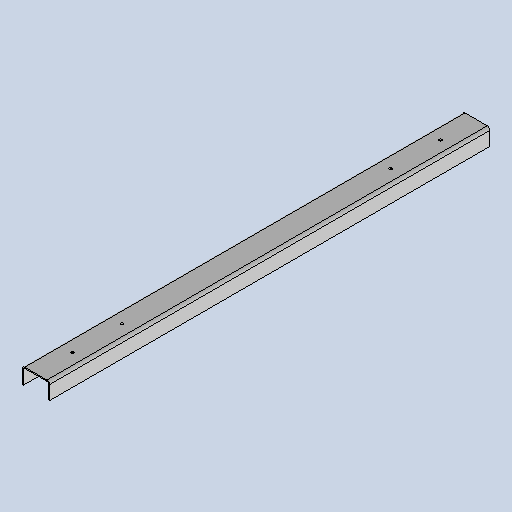
# Autodesk Inventor part: ДМФ 053 швеллер лотка v2.0_CPY
Saved by Autodesk Inventor 2026.2 (Build 302298010, 298A)
## iProperties
Created: 2024-05-13
Part Number: ДМФ 053 швеллер лотка v2.0_CPY
Material: Generic
Document SubType Name: Sheet Metal
Designer: admin
Mass: 164.292 g
Surface Area: 1680.29 cm^2
Volume: 164.292 cm^3
Density: 1 g/cm^3
Flat Pattern Width: 80 cm
Flat Pattern Length: 10.2404 cm
Flat Pattern Area: 819.232 cm^2
Sheet Metal Rule: Default
Sheet Metal Width: 800,000 mm
Sheet Metal Length: 102,404 mm
Sheet Metal Area: 81923,185 mm^2
Appearance: Default
Author: admin
Autodesk Inventor part; units mm, degrees
ref_plane "YZ Plane" through (0, 0, 0) normal (1, 0, 0) x (0, 1, 0)
ref_plane "XZ Plane" through (0, 0, 0) normal (0, 1, 0) x (-1, 0, 0)
ref_plane "XY Plane" through (0, 0, 0) normal (0, 0, 1) x (1, 0, 0)
sketch "Sketch1" plane through (0, 0, 0) normal (0, 0, 1) x (1, 0, 0)
  line L0 (-25, 0) -> (25, 0)
  line L1 (25, 0) -> (25, -800)
  line L2 (25, -800) -> (-25, -800)
  line L3 (-25, -800) -> (-25, 0)
  point P0 (0, 0)
  point P1 (0, 0)
  dimension "d0" = 50
  dimension "d1" = 800
  measures "d0" distance of L1.end L2.end
  measures "d1" distance of L0.end L1.end
extrude "Plate1" add sketch "Sketch1" along normal blind 2
sketch "Sketch2" plane through (23, -800, 2) normal (1, 0, 0) x (0, 1, 0)
  line L0 (800, 0) -> (0, 0)
  line L1 (0, 0) -> (0, -30)
  line L2 (0, -30) -> (800, -30)
  line L3 (800, -30) -> (800, 0)
  constraints: 6 end point, 1 horizontal, 1 perpendicular, 1 vertical
edge flange "Flange1" height 30 angle 90 thickness 2 bend radius 2.75 thickness toward (1, 0, 0) relief tear relief width 2 relief depth 1 corner gap 2 corner form 0 edges at (25, -400, 0) (-25, -400, 0) wall of the first edge with corners at (23, 0, 2) (23, -800, 2) (23, -800, -28) (23, 0, -28)
bend "Bend1"
corner "Corner1"
sketch "Sketch3" plane through (0, 0, 0) normal (1, 0, 0) x (0, 1, 0)
  line L0 (0, -2.75) -> (-800, -2.75) projected
  line L1 (-800, -28) -> (-800, -2.75) projected
  line L2 (0, -28) -> (-800, -28) projected
  line L3 (0, -2.75) -> (0, -28) projected
  line L4 (-790, -28) -> (-770, -28)
  line L5 (-770, -28) -> (-770, -18)
  line L6 (-770, -18) -> (-790, -18)
  line L7 (-790, -18) -> (-790, -28)
  point P0 (0, 0)
  point P1 (-770, -28)
  point P2 (-790, -23)
  dimension "d13" = 20
  dimension "d14" = 10
  dimension "d17" = 10
  constraints: 8 end point, 2 parallel, 1 horizontal, 1 midpoint, 1 perpendicular, 1 point on line
  measures "d13" distance of L6.end L5.end
  measures "d14" distance of L5.end L4.end
  measures "d17" distance from line of L1 point (-790, -23)
extrude "Extrusion1" [suppressed]
sketch "Sketch4" plane through (0, 0, 0) normal (0, 0, -1) x (-1, 0, 0)
  circle A0 centre (0, -733.4) radius 2.5
  circle A1 centre (0, -643.4) radius 2.5
  circle A2 centre (0, -155) radius 2.5
  circle A3 centre (0, -65) radius 2.5
  line L0 (20.25, 0) -> (-20.25, 0) projected
  line L1 (-20.25, 0) -> (20.25, 0) projected
  point P0 (0, 0)
  point P1 (0, 0)
  point P2 (0, 0)
  dimension "d18" = 5
  dimension "d19" = 90
  dimension "d20" = 90
  dimension "d21" = 488.4
  dimension "d22" = 65
  constraints: 4 centre point, 4 vertical alignment, 3 equal radius, 2 midpoint
  measures "d18" diameter of A0
  measures "d19" distance of A3.centre A2.centre
  measures "d20" distance of A1.centre A0.centre
  measures "d21" distance of A2.centre A1.centre
  measures "d22" distance of A3.centre point (0, 0)
extrude "Cut1" cut sketch "Sketch4" against normal blind 2
equation "\"d23\" = Thickness"
equation "\"d2\" = Thickness"
equation "\"d3\" = BendReliefWidth"
equation "\"d4\" = BendReliefDepth"
equation "\"d5\" = MinimumRemnant"
equation "\"d6\" = TransitionRadius"
equation "\"d10\" = CornerReliefSize"
equation "\"d11\" = GapSize"
equation "\"d12\" = JacobiRadiusSize"
equation "\"BendRadius\" = Thickness"
equation "\"BendReliefWidth\" = Thickness"
equation "\"BendReliefDepth\" = 0.5 * Thickness"
equation "\"CornerReliefSize\" = 4 * Thickness"
equation "\"MinimumRemnant\" = 2 * Thickness"
equation "\"TransitionRadius\" = BendRadius"
equation "\"JacobiRadiusSize\" = BendRadius"
equation "\"GapSize\" = Thickness"
equation "\"Thickness\" = 2"
body "Solid1"
